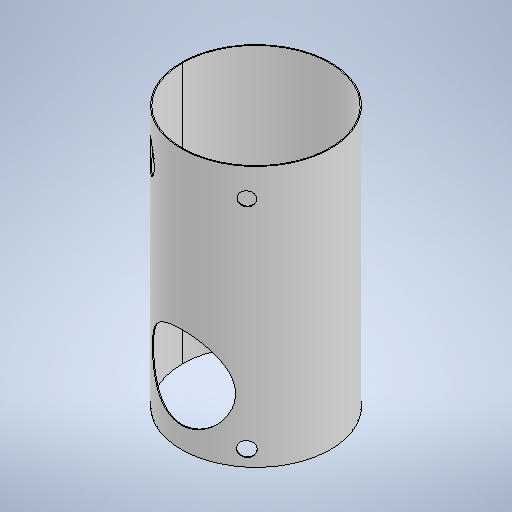
# Autodesk Inventor part: PNS-601 main tube D1000
Saved by Autodesk Inventor 2025 (Build 290162010, 162A)
## iProperties
Created: 2025-02-11
Part Number: PNS-601 main tube D1000
Material: Generic
Document SubType Name: Sheet Metal
Designer: pokla
Density: 1 g/cm^3
Flat Pattern Width: 166.23 cm
Flat Pattern Length: 296.886 cm
Flat Pattern Area: 49351.3 cm^2
Sheet Metal Rule: Default_mm
Sheet Metal Width: 1662,297 mm
Sheet Metal Length: 2968,860 mm
Sheet Metal Area: 4935126,451 mm^2
Appearance: Default
Author: pokla
Autodesk Inventor part; units mm, degrees
ref_plane "YZ Plane" through (0, 0, 0) normal (1, 0, 0) x (0, 1, 0)
ref_plane "XZ Plane" through (0, 0, 0) normal (0, 1, 0) x (-1, 0, 0)
ref_plane "XY Plane" through (0, 0, 0) normal (0, 0, 1) x (1, 0, 0)
sketch "Sketch1" plane through (0, 0, 0) normal (0, 1, 0) x (-1, 0, 0)
  line L0 (476, 1662.2969) -> (470, 1662.2969)
  line L1 (470, 1662.2969) -> (470, 0)
  line L2 (470, 0) -> (476, 0)
  line L3 (476, 0) -> (476, 1662.2969)
  line L4 (0, 0) -> (0, 1673.0415)
  point P0 (473, 0)
  dimension "d0" = 6
  dimension "d1" = 1662.2969
  dimension "d2" = 940
  constraints: 10 end point, 2 parallel, 1 coincident, 1 horizontal, 1 horizontal alignment, 1 midpoint, 1 perpendicular, 1 vertical
  measures "d0" distance between parallel lines of L1 L3
  measures "d1" distance of L2.end L0.start
  measures "d2" diameter of L1 L4
revolve "Revolution1" add sketch "Sketch1" angle 359.9 about axis through (0, 0, 0) along (0, 0, 1)
sketch "Sketch2" plane through (0, 0, 0) normal (0, 1, 0) x (-1, 0, 0)
  circle A0 centre (0, 400) radius 265
  line L0 (470, 1662.2969) -> (-470, 1662.2969) projected
  line L1 (110, 1462.2969) -> (-110, 1462.2969) construction
  line L2 (110, 1552.2969) -> (-110, 1552.2969)
  line L3 (-110, 1372.2969) -> (110, 1372.2969)
  arc A1 (110, 1372.2969) -> (110, 1552.2969) centre (110, 1462.2969) ccw
  arc A2 (-110, 1552.2969) -> (-110, 1372.2969) centre (-110, 1462.2969) ccw
  line L4 (200, 1462.2969) -> (-200, 1462.2969) construction
  point P0 (0, 0)
  point P1 (469.9993, 1662.2969)
  point P2 (0, 1462.2969)
  dimension "d4" = 530
  dimension "d12" = 400
  dimension "d15" = 200
  dimension "d16" = 400
  dimension "d17" = 180
  constraints: 10 end point, 6 point on circle, 4 tangent, 3 centre point, 2 vertical alignment, 1 horizontal, 1 midpoint, 1 parallel
  measures "d4" diameter of A0
  measures "d12" distance of A0.centre point (0, 0)
  measures "d15" distance between parallel lines of L1 L0
  measures "d16" distance of L4.start L4.end
  measures "d17" distance between parallel lines of L3 L2
extrude "Extrusion1" cut sketch "Sketch2" against normal through all contours A0
sketch "Sketch3" plane through (0, 0, 0) normal (0, 0, 1) x (1, 0, 0)
  line L0 (0, 0) -> (0, -267.717)
  line L1 (0, -267.717) -> (0, 0)
  line L2 (0, 0) -> (-206.5042, -173.2776)
  line L3 (0, 0) -> (-162.1162, -193.2026)
  dimension "d18" = 50
  dimension "d26" = 40
  constraints: 8 end point, 1 collinear, 1 vertical
  measures "d18" angle of L0 L2
  measures "d26" angle of L0 L3
ref_plane "Work Plane2" through (0, 0, -10) normal (0.6427876, -0.7660444, 0) x (0, 0, 1)
sketch "Sketch4" plane through (0, 0, -10) normal (0.6427876, -0.7660444, 0) x (0, 0, 1)
  circle A0 centre (1492.2969, 0) radius 45
  circle A1 centre (110, 0) radius 47.358
  line L0 (1672.2969, -476) -> (1672.2969, 476) projected
  point P0 (10, 0)
  point P1 (1672.2969, 364.6372)
  point P2 (1672.2969, 364.1026)
  dimension "d19" = 90
  dimension "d20" = 100
  dimension "d21" = 1482.2969
  dimension "d24" = 180
  constraints: 2 centre point, 2 horizontal alignment
  measures "d19" diameter of A0
  measures "d20" distance of A1.centre point (10, 0)
  measures "d21" distance of A0.centre point (10, 0)
  measures "d24" distance from line of L0 A0.centre
extrude "Extrusion2" cut sketch "Sketch4" along normal through all
ref_plane "Work Plane3" through (0, 0, 0) normal (-0.7660444, 0.6427876, 0) x (-0.6427876, -0.7660444, 0)
sketch "Sketch5" plane through (0, 0, 0) normal (-0.7660444, 0.6427876, 0) x (-0.6427876, -0.7660444, 0)
  line L0 (476, 1662.2969) -> (-476, 1662.2969) projected
  line L1 (476, 1412.2969) -> (0, 1137.4782)
  point P0 (0, 0)
  point P1 (305.9669, 1662.2969)
  point P2 (305.33, 1662.2969)
  point P3 (0, 1662.2969)
  dimension "d27" = 30
  dimension "d28" = 250
  constraints: 2 end point, 1 midpoint, 1 vertical alignment
  measures "d27" angle of L0 L1
  measures "d28" distance from line of L0 L1.start
ref_plane "Work Plane4" through (0, 0, 1137.4782) normal (0.5566704, 0.6634139, -0.5) x (-0.7660444, 0.6427876, 0)
sketch "Sketch6" plane through (0, 0, 1137.4782) normal (0.5566704, 0.6634139, -0.5) x (-0.7660444, 0.6427876, 0)
  circle A0 centre (0, 0) radius 85
  point P0 (0, -985.085)
  point P1 (0, 0)
  dimension "d29" = 170
  constraints: 1 centre point, 1 coincident
  measures "d29" diameter of A0
extrude "Extrusion3" cut sketch "Sketch6" against normal through all
equation "\"d1\" = MAIN_hight - 2 * Disherd_head_hight"
equation "\"d2\" = MAIN_filter_diam"
equation "\"d4\" = Accsess_hatch_diameter"
equation "\"d16\" = Charging_hatch_width"
equation "\"d17\" = Charging_hatch_hight"
equation "\"BendRadius\" = Thickness"
equation "\"BendReliefWidth\" = Thickness"
equation "\"BendReliefDepth\" = 0.5 * Thickness"
equation "\"CornerReliefSize\" = 4 * Thickness"
equation "\"MinimumRemnant\" = 2 * Thickness"
equation "\"TransitionRadius\" = BendRadius"
equation "\"JacobiRadiusSize\" = BendRadius"
equation "\"GapSize\" = Thickness"
equation "\"MAIN_hight\" = 2100"
equation "\"Disherd_head_hight\" = 218.851546"
equation "\"MAIN_filter_diam\" = 940"
equation "\"Accsess_hatch_diameter\" = 530"
equation "\"Charging_hatch_width\" = 400"
equation "\"Charging_hatch_hight\" = 180"
equation "\"Thickness\" = 6"
body "Solid1"
